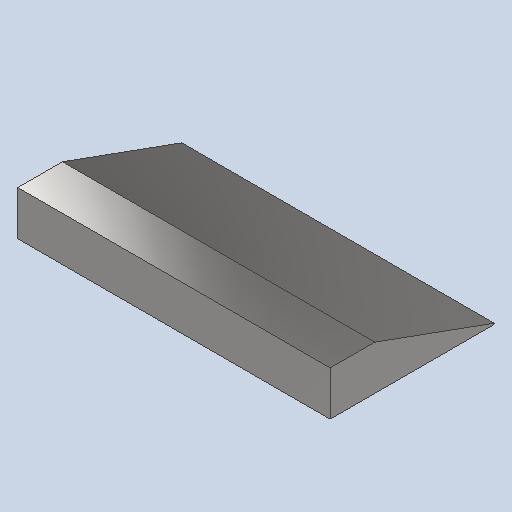
# Autodesk Inventor part: body_flaps
Saved by Autodesk Inventor 2024 (Build 280153000, 153)
## iProperties
Created: 2023-06-07
Part Number: body_flaps
Material: Steel, Mild
Document SubType Name: Modeling
Designer: tamiz
Density: 7.85 g/cm^3
Appearance: Semi-Polished
Author: tamiz
Autodesk Inventor part; units mm, degrees
ref_plane "YZ Plane" through (0, 0, 0) normal (1, 0, 0) x (0, 1, 0)
ref_plane "XZ Plane" through (0, 0, 0) normal (0, 1, 0) x (-1, 0, 0)
ref_plane "XY Plane" through (0, 0, 0) normal (0, 0, 1) x (1, 0, 0)
sketch "Sketch1" plane through (0, 0, 0) normal (0, 1, 0) x (-1, 0, 0)
  line L0 (0, 0) -> (6400.8, 0)
  line L1 (6400.8, 0) -> (6400.8, -3352.8)
  line L2 (6400.8, -3352.8) -> (0, -3352.8)
  line L3 (0, -3352.8) -> (0, 0)
  dimension "d0" = 6400.8
  dimension "d1" = 3352.8
  constraints: 8 end point, 2 parallel, 1 horizontal, 1 perpendicular
  measures "d0" distance of L1.end L2.end
  measures "d1" distance of L0.end L1.end
extrude "Extrusion1" add sketch "Sketch1" along normal blind 25.4
sketch "Sketch2" plane through (0, 25.4, 0) normal (0, 1, 0) x (1, 0, 0)
  line L0 (-6400.8, 3352.8) -> (-6400.8, 0) projected
  line L1 (-6400.8, 0) -> (0, 0)
  line L2 (0, 0) -> (0, 914.4)
  line L3 (0, 914.4) -> (-6400.8, 914.4)
  line L4 (-6400.8, 914.4) -> (-6400.8, 0)
  dimension "d4" = 6400.8
  dimension "d5" = 914.4
  constraints: 8 end point, 2 parallel, 1 horizontal, 1 perpendicular
  measures "d4" distance of L3.end L2.end
  measures "d5" distance of L2.end L1.end
extrude "Extrusion2" add sketch "Sketch2" along normal blind 883.92
ref_plane "Work Plane1" through (0, 25.4, -3352.8) normal (0, 0.9401361, -0.3407993) x (-1, 0, 0)
sketch "Sketch3" plane through (0, 25.4, -3352.8) normal (0, 0.9401361, -0.3407993) x (-1, 0, 0)
  line L0 (0, 3143.4319) -> (0, -8.6563) projected
  line L1 (0, 2593.6671) -> (6400.8, 2593.6671) projected
  line L2 (0, -8.6563) -> (6400.8, -8.6563)
  line L3 (6400.8, -8.6563) -> (6400.8, 2593.6671)
  line L4 (6400.8, 2593.6671) -> (0, 2593.6671)
  line L5 (0, 2593.6671) -> (0, -8.6563)
  constraints: 8 end point, 2 parallel, 1 horizontal, 1 perpendicular
extrude "Extrusion3" add sketch "Sketch3" against normal through all
body "Solid1"
